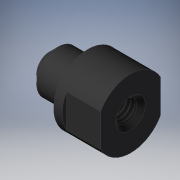
# Autodesk Inventor part: URLM8_c
Saved by Autodesk Inventor 2019 (Build 230136000, 136)
## iProperties
Created: 2024-01-11
Part Number: URLM8_c
Material: Generic
Catalog Web Link: www.cadenas.de
Description: URLH, URLM, URLL_core_rod-Urethane Pushers -Tapped - Flat
Vendor: MISUMI
Document SubType Name: Modeling
Designer: psAdmin
Manufacturer: MISUMI
Mass: 0.283197 g
Surface Area: 3.43996 cm^2
Volume: 0.283197 cm^3
Density: 1 g/cm^3
Appearance: PSOLRGB-175-175-175
Category: PARTsolutions
Company: MISUMI
Title: URLM8
Author: Cadenas PARTsolutions
Comments: Urethane Pushers -Tapped - Flat
PSOL_IDENT_0: {$CADENAS_DATA/23d-libs/misumi/metric/34_cylinders/urlh_core_rod.prj},182 {VTYP=3D},{NB=URLM8_c},{LI
PSOL_IDENT_1: NA=URLM8},{NN=URLH, URLM, URLL_core_rod},{DATE=04.06.2021 00:06:22},{GEOMDATE=17.02.2014 00:00:00},{
PSOL_IDENT_2: VERSION=},{LINEID=10},{WBVAR=MATP,HARD,M},{WBNUMERIC=}  {NB=URLM8_c},{LINA=URLM8},{KT=DUMMY},{PN=URL
PSOL_IDENT_3: M8},{TYPE=URLM},{MATCR=304 Stainless Steel},{MATP=2},{MATP1='1', 'Ether Type Polyurethane', '2', 'Es
PSOL_IDENT_4: ter Type Polyurethane'},{HARD=2},{HARD0='2', 'Shore A70','3','Shore A50'},{D=8},{L=12},{M=1},{M1=3},
PSOL_IDENT_5: {MALG='1','M3x0.5'},{SR1=8},{R2=1.0},{LL1=5},{LL2=4},{W=7},{NDM=5},{KDM=2.459},{P=0.50},{ALG=},{UH=8
PSOL_IDENT_6: .5},{CR1=9.5},{CRC=1},{CRC1=0.5}
NB: URLM8_c
NN: URLH, URLM, URLL_core_rod
NT: Urethane Pushers -Tapped - Flat
NBSYN: $PN._c
LINA: URLM8
CATALOG: Misumi
PN: URLM8
MATCR: 304 Stainless Steel
MATP: Ester Type Polyurethane
HARD: Shore A70
D: 8
L: 12
M: M3x0.5
SR1: 8
R2: 1
LL1: 5
LL2: 4
W: 7
SUPPLIER: MISUMI
ARTICLENO: URLM8_c
BOMINFO: URLM8
CREATOR: CADENAS GmbH
Autodesk Inventor part; units mm, degrees
sketch "Sketch_1" plane through (0, 0, 0) normal (0, 0, 1) x (1, 0, 0)
  line L0 (9.5, 0) -> (0, 0)
  line L1 (0, 0) -> (0, 1.5)
  line L2 (0, 1.5) -> (1, 2.5)
  line L3 (1, 2.5) -> (4.5, 2.5)
  line L4 (4.5, 2.5) -> (4.5, 4)
  line L5 (4.5, 4) -> (9.5, 4)
  line L6 (9.5, 4) -> (9.5, 0)
  line L7 (9.5, 0) -> (0, 0)
  constraints: 16 end point
revolve "Revolution1" add sketch "Sketch_1" angle 360 about axis through (9.5, 0, 0) along (1, 0, 0)
sketch "Sketch2" plane through (9.5, 0, 0) normal (1, 0, 0) x (0, 0, -1)
  point P0 (0, 0)
hole "Hole1" at (9.5, 0, 0) direction (-1, 0, 0) diameter 2.459 depth 7.7901 tip angle 120 countersink diameter 3.459 countersink angle 90 thread size "M3x0.5" class "6H" standard "ISO Metric profile"
sketch "Sketch_2" plane through (9.5, 0, 0) normal (1, 0, 0) x (0, 0, -1)
  line L0 (-7, 7) -> (-7, -7)
  line L1 (-7, -7) -> (7, -7)
  line L2 (7, -7) -> (7, 7)
  line L3 (7, 7) -> (-7, 7)
  line L4 (-3.5, 1.9571) -> (-3.5, -1.9571)
  arc A0 (-3.5, -1.9571) -> (3.5, -1.9571) centre (0, 0) ccw
  line L5 (3.5, -1.9571) -> (3.5, 1.9571)
  arc A1 (3.5, 1.9571) -> (-3.5, 1.9571) centre (0, 0) ccw
  constraints: 12 end point, 4 point on circle, 2 centre point
extrude "Extrusion1" cut sketch "Sketch_2" against normal blind 4
ref_plane "core_rod_XY" through (4.5, 0, 0) normal (1, 0, 0) x (0, 0, -1)
ref_plane "core_rod_YZ" through (4.5, 0, 0) normal (0, 0, -1) x (0, 1, 0)
ref_plane "core_rod_ZX" through (4.5, 0, 0) normal (0, 1, 0) x (1, 0, 0)
body "Solid1"
